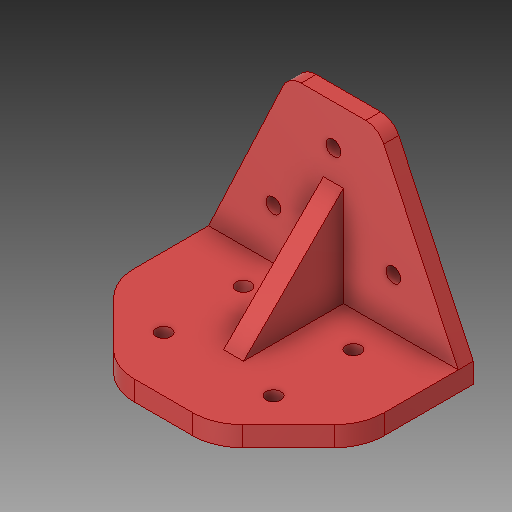
# Autodesk Inventor part: Wspornik
Saved by Autodesk Inventor 2018 (Build 220112000, 112)
## iProperties
Created: 2018-08-13
Part Number: Wspornik
Material: Tworzywo sztuczne PET
Document SubType Name: Modeling
Designer: Wojciech
Density: 1.541 g/cm^3
Appearance: Gładki - czerwony
Mass: 16.2579 g
Surface Area: 67.7512 cm^2
Volume: 10.5502 cm^3
Author: Wojciech
Autodesk Inventor part; units mm, degrees
ref_plane "YZ Plane" through (0, 0, 0) normal (1, 0, 0) x (0, 1, 0)
ref_plane "XZ Plane" through (0, 0, 0) normal (0, 1, 0) x (-1, 0, 0)
ref_plane "XY Plane" through (0, 0, 0) normal (0, 0, 1) x (1, 0, 0)
sketch "Szkic1" plane through (0, 0, 0) normal (0, 1, 0) x (-1, 0, 0)
  line L0 (25, 19) -> (-25, 19)
  line L1 (-25, 19) -> (-25, -19)
  line L2 (-25, -19) -> (25, -19)
  line L3 (25, -19) -> (25, 19)
  line L4 (25, 19) -> (-25, -19) construction
  line L5 (-25, 19) -> (25, -19) construction
  point P0 (0, 0)
  dimension "d0" = 50
  dimension "d1" = 38
  constraints: 12 end point, 2 midpoint, 2 parallel, 1 horizontal, 1 perpendicular
  measures "d0" distance of L2.end L1.end
  measures "d1" distance of L1.end L0.end
extrude "Wyciągnięcie proste1" add sketch "Szkic1" along normal blind 4
sketch "Szkic2" plane through (0, 4, 0) normal (0, 1, 0) x (1, 0, 0)
  line L0 (-25, 19) -> (-25, -19) projected
  line L1 (25, -19) -> (25, 19) projected
  line L2 (-25, 19) -> (25, 19)
  line L3 (25, 19) -> (25, 15)
  line L4 (25, 15) -> (-25, 15)
  line L5 (-25, 15) -> (-25, 19)
  point P0 (0, 0)
  dimension "d4" = 4
  constraints: 8 end point, 2 parallel, 1 horizontal, 1 perpendicular, 1 point on line
  measures "d4" distance of L2.end L3.end
extrude "Wyciągnięcie proste2" add sketch "Szkic2" along normal blind 34
sketch "Szkic3" plane through (0, 4, 0) normal (0, 1, 0) x (1, 0, 0)
  line L0 (25, -19) -> (25, 19) projected
  line L1 (25, 0) -> (-25, 0) construction
  line L2 (-25, 19) -> (-25, -19) projected
  line L3 (-25, 15) -> (25, 15) projected
  line L4 (0, 15) -> (0, -19) construction
  line L5 (0, -15) -> (0, 19) construction
  point P0 (0, 0)
  point P1 (-11, 8)
  point P2 (-11, -8)
  point P3 (11, 8)
  point P4 (11, -8)
  dimension "d7" = 8
  dimension "d8" = 11
  constraints: 6 end point, 5 symmetric about line, 3 midpoint, 1 vertical
  measures "d7" distance from line of L1 point (-11, 8)
  measures "d8" distance from line of L4 point (-11, 8)
hole "Otwór1" at (-11, 4, -8) at (-11, 4, 8) at (11, 4, 8) at (11, 4, -8) direction (0, -1, 0) diameter 3 depth 8 tip angle 118
sketch "Szkic4" plane through (-25, 4, -15) normal (0, 0, 1) x (1, 0, 0)
  line L0 (50, 34) -> (0, 34) projected
  line L1 (0, 0) -> (0, 34) projected
  line L2 (50, 0) -> (0, 0) projected
  line L3 (25, 34) -> (25, 0) construction
  point P0 (25, -4)
  point P1 (25, 26)
  point P2 (13, 10)
  point P3 (37, 10)
  dimension "d16" = 8
  dimension "d17" = 25
  dimension "d18" = 13
  dimension "d19" = 10
  constraints: 2 end point, 2 midpoint, 1 symmetric about line
  measures "d16" distance from line of L0 point (25, 26)
  measures "d17" distance from line of L1 point (25, 26)
  measures "d18" distance from line of L1 point (13, 10)
  measures "d19" distance from line of L2 point (13, 10)
hole "Otwór2" at (0, 30, -15) at (-12, 14, -15) at (12, 14, -15) direction (0, 0, -1) diameter 3 depth 8 tip angle 118
sketch "Szkic5" plane through (-25, 4, -15) normal (0, 0, 1) x (1, 0, 0)
  line L0 (0, 34) -> (50, 34) projected
  line L1 (50, 0) -> (50, 34) projected
  line L2 (50, 0) -> (0, 0) projected
  line L3 (34, 34) -> (50, 0)
  line L4 (34, 34) -> (50, 34)
  line L5 (50, 34) -> (50, 0)
  line L6 (25, 34) -> (25, 0) construction
  line L7 (50, 34) -> (0, 34)
  line L8 (0, 0) -> (0, 34)
  line L9 (0, 0) -> (50, 0)
  line L10 (16, 34) -> (0, 0)
  line L11 (16, 34) -> (0, 34)
  line L12 (0, 34) -> (0, 0)
  point P0 (25, -4)
  dimension "d27" = 16
  constraints: 20 end point, 5 symmetric about line, 2 collinear, 2 midpoint, 2 point on line
  measures "d27" distance from line of L1 L3.start
extrude "Wyciągnięcie proste3" cut sketch "Szkic5" against normal blind 34 contours L0 L10 L8 | L0 L1 L3
fillet "Zaokrąglenie1" radius 4 2 edges at (-9, 38, -17) (9, 38, -17)
sketch "Szkic7" plane through (0, 4, 0) normal (0, 1, 0) x (1, 0, 0)
  line L0 (25, 15) -> (-25, 15) projected
  line L1 (-2, 15) -> (2, 15)
  line L2 (2, 15) -> (2, -5)
  line L3 (2, -5) -> (-2, -5)
  line L4 (-2, -5) -> (-2, 15)
  point P0 (0, 0)
  dimension "d31" = 4
  dimension "d32" = 20
  dimension "d33" = 2
  constraints: 8 end point, 2 parallel, 1 horizontal, 1 perpendicular, 1 point on line
  measures "d31" distance of L2.end L3.end
  measures "d32" distance of L1.end L2.end
  measures "d33" distance from line of point (0, 0) L4
extrude "Wyciągnięcie proste4" add sketch "Szkic7" along normal blind 20
sketch "Szkic8" plane through (2, 4, 5) normal (1, 0, 0) x (0, 0, -1)
  line L0 (20, 20) -> (0, 20) projected
  line L1 (20, 20) -> (0, 0)
  line L2 (0, 0) -> (0, 20)
  line L3 (-14, -4) -> (24, -4) projected
  line L4 (0, 20) -> (20, 20)
  point P0 (5, -4)
  constraints: 6 end point, 2 perpendicular
extrude "Wyciągnięcie proste5" cut sketch "Szkic8" against normal blind 18
sketch "Szkic9" plane through (25, 0, 19) normal (1, 0, 0) x (0, 0, -1)
  line L0 (38, 0) -> (0, 0) projected
  line L1 (38, 0) -> (37, 0)
  line L2 (37, 0) -> (37, 38)
  line L3 (37, 38) -> (38, 38)
  line L4 (38, 38) -> (38, 0)
  point P0 (19, 0)
  dimension "d38" = 1
  dimension "d39" = 38
  constraints: 8 end point, 2 parallel, 1 horizontal, 1 perpendicular
  measures "d38" distance of L2.end L3.end
  measures "d39" distance of L1.end L2.end
extrude "Wyciągnięcie proste6" cut sketch "Szkic9" against normal through all
chamfer "Faza1" distance 15 angle 45 2 edges at (25, 2, 19) (-25, 2, 19)
fillet "Zaokrąglenie2" radius 10 4 edges at (25, 2, 4) (10, 2, 19) (-10, 2, 19) (-25, 2, 4)
